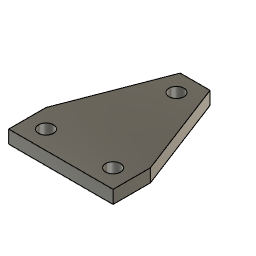
CoverSlip (Autodesk Fusion 360 design; units mm, degrees)
Autodesk Fusion 360 part; units mm, degrees
sketch "windowThroughHoles" plane through (0, 0, 0) normal (0, 0, 1) x (1, 0, 0)
  line L0 (0, 0) -> (14, 0)
  line L1 (0, 5) -> (5, 18)
  circle A0 centre (7, 15.5) radius 1
  circle A1 centre (2.5, 2.5) radius 1
  circle A2 centre (11.5, 2.5) radius 1
  line L2 (14, 18) -> (0, 18)
  line L3 (0, 18) -> (0, 0)
  line L4 (5, 18) -> (9, 18)
  line L5 (0, 0) -> (0, 5)
  line L6 (14, 5) -> (9, 18)
  line L7 (0, 0) -> (14, 0)
  line L8 (14, 0) -> (14, 5)
  line L9 (14, 0) -> (14, 18)
  dimension "d1" = 13
  dimension "d2" = 4.5
  dimension "d3" = 13
  dimension "d4" = 4.5
  dimension "d5" = 18
  dimension "d6" = 14
  dimension "d7" = 13.9284
  dimension "d8" = 13.9284
  dimension "d9" = 4
  dimension "d10" = 2
  measures "d1" vertical distance of A0.centre A2.centre
  measures "d2" horizontal distance of A0.centre A2.centre
  measures "d3" vertical distance of A0.centre A1.centre
  measures "d4" horizontal distance of A0.centre A1.centre
  measures "d5" distance of L0 L2
  measures "d6" distance of L3 L9
  measures "d7" distance of L1.start L1.end
  measures "d8" distance of L4.end L6.start
  measures "d9" distance of L1.end L4.end
  measures "d10" diameter of A2
extrude "Extrude1" add sketch "windowThroughHoles" along normal blind 1.7526 contours L0 L1 L2 L3 L4 L5 L6 L7 L8 L9
